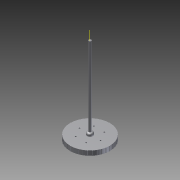
# Autodesk Inventor part: Stand
Saved by Autodesk Inventor 2012 SP2 (Build 160219200, 219)
## iProperties
Created: 2014-02-06
Part Number: Stand
Material: Default
Document SubType Name: Modeling
Designer: 1
Density: 1 g/cm^3
Author: 1
Autodesk Inventor part; units mm, degrees
ref_plane "YZ Plane" through (0, 0, 0) normal (1, 0, 0) x (0, 1, 0)
ref_plane "XZ Plane" through (0, 0, 0) normal (0, 1, 0) x (-1, 0, 0)
ref_plane "XY Plane" through (0, 0, 0) normal (0, 0, 1) x (1, 0, 0)
ref_plane "Work Plane1" through (0, 0, 0) normal (0, 1, 0) x (-1, 0, 0)
sketch "Sketch2" plane through (0, 0, 0) normal (0, 1, 0) x (-1, 0, 0)
  circle A0 centre (0, 0) radius 150
  dimension "d2" = 300
  constraints: 1 centre point, 1 coincident
  measures "d2" diameter of A0
extrude "Extrusion1" add sketch "Sketch2" along normal blind 35
sketch "Sketch3" plane through (0, 35, 0) normal (0, 1, 0) x (1, 0, 0)
  circle A0 centre (0, 0) radius 150 projected
  circle A1 centre (-150, 0) radius 2
  line L0 (0, 0) -> (-150, 0) construction
  dimension "d5" = 4
  constraints: 2 end point, 1 centre point, 1 horizontal, 1 horizontal alignment, 1 other
  measures "d5" diameter of A1
extrude "Extrusion2" add sketch "Sketch3" against normal up to surface (35 mm away) contours A1 A0 | A0 A1 picked at (-149.3323, 0) picked at (-150.6608, 0.0807)
pattern_circular "Circular Pattern1" count 36 over 360 about axis through (0, -10, 0) along (0, 1, 0) of "Extrusion2"
sketch "Sketch4" plane through (0, 35, 0) normal (0, 1, 0) x (1, 0, 0)
  arc A0 (-141.6254, 49.4191) -> (-147.3607, 28.0145) centre (0, 0) ccw projected
  circle A1 centre (0, 0) radius 22.0533
  constraints: 1 centre point, 1 coincident
extrude "Extrusion3" add sketch "Sketch4" along normal blind 20
sketch "Sketch5" plane through (0, 55, 0) normal (0, 1, 0) x (1, 0, 0)
  circle A0 centre (0, 0) radius 22.0533 projected
  circle A1 centre (0, 0) radius 10
  dimension "d13" = 20
  constraints: 1 centre point, 1 coincident
  measures "d13" diameter of A1
extrude "Extrusion4" add sketch "Sketch5" along normal blind 600 contours A1
fillet "Fillet1" radius 11.525 1 edges at (-22.0533, 55, 0)
sketch "Sketch6" plane through (0, 35, 0) normal (0, 1, 0) x (1, 0, 0)
  circle A0 centre (0, 0) radius 22.0533 projected
  circle A1 centre (-80, 0) radius 5
  dimension "d17" = 80
  dimension "d18" = 10
  constraints: 1 centre point
  measures "d17" distance of A0.centre A1.centre
  measures "d18" diameter of A1
extrude "Extrusion5" cut sketch "Sketch6" against normal through all contours A1
pattern_circular "Circular Pattern2" count 6 over 360 about axis through (0, -10, 0) along (0, 1, 0) of "Extrusion5"
body "Solid1"
